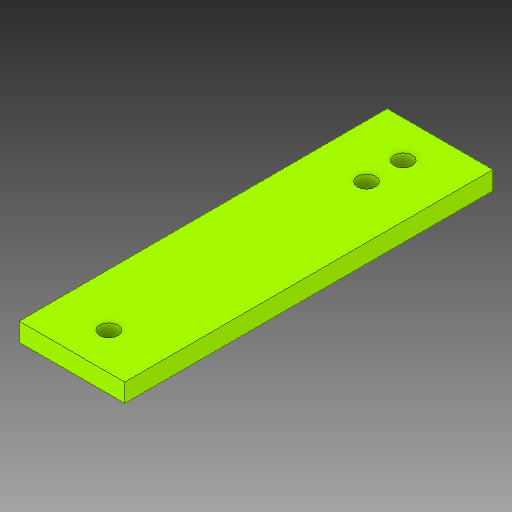
# Autodesk Inventor part: plat
Saved by Autodesk Inventor 2018 (Build 220112000, 112)
## iProperties
Created: 2019-12-19
Part Number: plat
Material: Generic
Document SubType Name: Modeling
Designer: Ibnu
Density: 1 g/cm^3
Appearance: Default
Author: Ibnu
Autodesk Inventor part; units mm, degrees
ref_plane "YZ Plane" through (0, 0, 0) normal (1, 0, 0) x (0, 1, 0)
ref_plane "XZ Plane" through (0, 0, 0) normal (0, 1, 0) x (-1, 0, 0)
ref_plane "XY Plane" through (0, 0, 0) normal (0, 0, 1) x (1, 0, 0)
sketch "Sketch1" plane through (0, 0, 0) normal (0, 1, 0) x (-1, 0, 0)
  line L0 (14.35, -100) -> (-14.35, -100)
  line L1 (14.35, 0) -> (14.35, -100)
  line L2 (14.35, 0) -> (-14.35, 0)
  line L3 (14.35, 0) -> (-14.35, 0)
  line L4 (-14.35, -100) -> (-14.35, 0)
  point P0 (0, 0)
  constraints: 10 end point, 1 collinear, 1 horizontal, 1 perpendicular, 1 vertical
extrude "Extrusion1" add sketch "Sketch1" along normal blind 5
sketch "Sketch2" plane through (0, 5, 0) normal (0, 1, 0) x (1, 0, 0)
  circle A0 centre (0, 80) radius 2.5
  circle A1 centre (0, 90) radius 2.5
  circle A2 centre (0, 10) radius 2.5
  point P0 (0, 0)
  constraints: 3 centre point
extrude "Extrusion2" cut sketch "Sketch2" against normal through all
body "Solid1"
